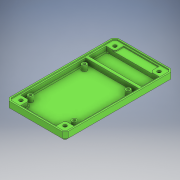
# Autodesk Inventor part: Case2
Saved by Autodesk Inventor 2020 (Build 240168000, 168)
## iProperties
Created: 2020-11-28
Part Number: Case2
Material: PBT Plastic
Document SubType Name: Modeling
Designer: Milosz
Density: 1.31 g/cm^3
Appearance: Smooth - White
Author: Milosz
## iProperties of the stored document _3DPrint.ipt
Created: 2020-11-29
Part Number: _3DPrint
Material: Generic
Document SubType Name: Modeling
Designer: Milosz
Density: 1 g/cm^3
Appearance: Default
Author: Milosz
Autodesk Inventor part; units mm, degrees
ref_plane "YZ Plane" through (0, 0, 0) normal (1, 0, 0) x (0, 1, 0)
ref_plane "XZ Plane" through (0, 0, 0) normal (0, 1, 0) x (-1, 0, 0)
ref_plane "XY Plane" through (0, 0, 0) normal (0, 0, 1) x (1, 0, 0)
sketch "Sketch4" plane through (0, 0, 0) normal (0, 1, 0) x (-1, 0, 0)
  circle A0 centre (-31.1, -7.3) radius 1.75
  line L0 (-34.858, -107.35) -> (16.858, -107.35)
  line L1 (16.858, -107.35) -> (18.95, -105.258)
  line L2 (18.95, -105.258) -> (18.95, -3.542)
  line L3 (18.95, -3.542) -> (16.858, -1.45)
  line L4 (16.858, -1.45) -> (-34.858, -1.45)
  line L5 (-34.858, -1.45) -> (-36.95, -3.542)
  line L6 (-36.95, -3.542) -> (-36.95, -105.258)
  line L7 (-36.95, -105.258) -> (-34.858, -107.35)
  circle A1 centre (-31.1, -101.5) radius 1.75
  circle A2 centre (13.1, -7.3) radius 1.75
  line L8 (8.7, -99.1) -> (10.7, -97.1)
  line L9 (8.7, -99.1) -> (8.7, -105.9)
  line L10 (8.7, -105.9) -> (-26.7, -105.9)
  line L11 (-26.7, -99.1) -> (-26.7, -105.9)
  line L12 (-28.7, -97.1) -> (-26.7, -99.1)
  line L13 (-35.5, -97.1) -> (-28.7, -97.1)
  line L14 (-35.5, -97.1) -> (-35.5, -11.7)
  line L15 (-35.5, -11.7) -> (-28.7, -11.7)
  line L16 (-26.7, -9.7) -> (-28.7, -11.7)
  line L17 (-26.7, -9.7) -> (-26.7, -2.9)
  line L18 (-26.7, -2.9) -> (8.7, -2.9)
  line L19 (8.7, -9.7) -> (8.7, -2.9)
  line L20 (10.7, -11.7) -> (8.7, -9.7)
  line L21 (17.5, -11.7) -> (10.7, -11.7)
  line L22 (17.5, -11.7) -> (17.5, -97.1)
  line L23 (17.5, -97.1) -> (10.7, -97.1)
  circle A3 centre (13.1, -101.5) radius 1.75
  line L24 (20.5, -2.9) -> (20.5, -105.9)
  line L25 (17.5, 0.1) -> (20.5, -2.9)
  line L26 (-35.5, 0.1) -> (17.5, 0.1)
  line L27 (-38.5, -2.9) -> (-35.5, 0.1)
  line L28 (-38.5, -105.9) -> (-38.5, -2.9)
  line L29 (-35.5, -108.9) -> (-38.5, -105.9)
  line L30 (17.5, -108.9) -> (-35.5, -108.9)
  line L31 (20.5, -105.9) -> (17.5, -108.9)
  line L32 (16.858, -107.35) -> (18.95, -105.258)
  line L33 (-34.858, -107.35) -> (16.858, -107.35)
  line L34 (-36.95, -105.258) -> (-34.858, -107.35)
  line L35 (-36.95, -3.542) -> (-36.95, -105.258)
  line L36 (-34.858, -1.45) -> (-36.95, -3.542)
  line L37 (16.858, -1.45) -> (-34.858, -1.45)
  line L38 (18.95, -3.542) -> (16.858, -1.45)
  line L39 (18.95, -105.258) -> (18.95, -3.542)
  line L40 (-37.05, -105.2994) -> (-37.05, -3.5006)
  line L41 (-37.05, -3.5006) -> (-34.8994, -1.35)
  line L42 (-34.8994, -1.35) -> (16.8994, -1.35)
  line L43 (16.8994, -1.35) -> (19.05, -3.5006)
  line L44 (19.05, -3.5006) -> (19.05, -105.2994)
  line L45 (19.05, -105.2994) -> (16.8994, -107.45)
  line L46 (16.8994, -107.45) -> (-34.8994, -107.45)
  line L47 (-34.8994, -107.45) -> (-37.05, -105.2994)
  point P0 (0, 0)
  point P1 (0, 0)
  dimension "d29" = 0.1
  constraints: 96 end point, 4 centre point, 7 other
  measures "d29" distance between parallel lines of L6 L40
extrude "Extrusion3" add sketch "Sketch4" along normal blind 1 contours L24 L31 L30 L29 L28 L27 L26 L25
extrude "Extrusion4" add sketch "Sketch4" against normal blind 5 contours L7 L6 L5 L4 L3 L2 L1 L0 | L24 L31 L30 L29 L28 L27 L26 L25 | L40 L41 L42 L43 L44 L45 L46 L47
sketch "Sketch5" plane through (0, -5, 0) normal (0, -1, 0) x (1, 0, 0)
  line L0 (38.5, -105.9) -> (38.5, -2.9) projected
  line L1 (38.5, -2.9) -> (35.5, 0.1) projected
  line L2 (35.5, 0.1) -> (-17.5, 0.1) projected
  line L3 (35.5, 0.1) -> (-17.5, 0.1) projected
  line L4 (-17.5, 0.1) -> (-20.5, -2.9) projected
  line L5 (-20.5, -2.9) -> (-20.5, -105.9) projected
  line L6 (-20.5, -105.9) -> (-17.5, -108.9) projected
  line L7 (-17.5, -108.9) -> (35.5, -108.9) projected
  line L8 (35.5, -108.9) -> (38.5, -105.9) projected
  line L9 (38.5, -105.9) -> (38.5, -2.9) projected
  line L10 (38.5, -2.9) -> (35.5, 0.1) projected
  circle A0 centre (31.1, -101.5) radius 1.75 projected
  circle A1 centre (-13.1, -101.5) radius 1.75 projected
  circle A2 centre (31.1, -7.3) radius 1.75 projected
  circle A3 centre (-13.1, -7.3) radius 1.75 projected
  line L11 (-17.5, -11.7) -> (-10.7, -11.7) projected
  line L12 (-10.7, -11.7) -> (-8.7, -9.7) projected
  line L13 (-8.7, -9.7) -> (-8.7, -2.9) projected
  line L14 (-8.7, -2.9) -> (26.7, -2.9) projected
  line L15 (26.7, -2.9) -> (26.7, -9.7) projected
  line L16 (26.7, -9.7) -> (28.7, -11.7) projected
  line L17 (28.7, -11.7) -> (35.5, -11.7) projected
  line L18 (35.5, -11.7) -> (35.5, -97.1) projected
  line L19 (35.5, -97.1) -> (28.7, -97.1) projected
  line L20 (28.7, -97.1) -> (26.7, -99.1) projected
  line L21 (26.7, -99.1) -> (26.7, -105.9) projected
  line L22 (26.7, -105.9) -> (-8.7, -105.9) projected
  line L23 (-8.7, -105.9) -> (-8.7, -99.1) projected
  line L24 (-8.7, -99.1) -> (-10.7, -97.1) projected
  line L25 (-10.7, -97.1) -> (-17.5, -97.1) projected
  line L26 (-17.5, -97.1) -> (-17.5, -11.7) projected
  point P0 (0, 0)
extrude "Extrusion5" add sketch "Sketch5" along normal blind 3 contours L8 L7 L6 L5 L4 L2 L1 L0 | L11 L12 L13 L14 L15 L16 L17 L18 L19 L20 L21 L22 L23 L24 L25 L26
sketch "Sketch6" plane through (0, -8, 0) normal (0, -1, 0) x (1, 0, 0)
  line L0 (38.5, -2.9) -> (35.5, 0.1) projected
  line L1 (35.5, 0.1) -> (-17.5, 0.1) projected
  line L2 (-17.5, 0.1) -> (-20.5, -2.9) projected
  line L3 (-20.5, -2.9) -> (-20.5, -105.9) projected
  line L4 (-20.5, -105.9) -> (-17.5, -108.9) projected
  line L5 (-17.5, -108.9) -> (35.5, -108.9) projected
  line L6 (35.5, -108.9) -> (38.5, -105.9) projected
  line L7 (38.5, -105.9) -> (38.5, -2.9) projected
  circle A0 centre (31.1, -101.5) radius 1.75 projected
  circle A1 centre (-13.1, -101.5) radius 1.75 projected
  circle A2 centre (31.1, -7.3) radius 1.75 projected
  circle A3 centre (-13.1, -7.3) radius 1.75 projected
  circle A4 centre (31.1, -7.3) radius 3
  circle A5 centre (31.1, -101.5) radius 3
  circle A6 centre (-13.1, -101.5) radius 3
  circle A7 centre (-13.1, -7.3) radius 3
  point P0 (0, 0)
  dimension "d17" = 6
  dimension "d18" = 6
  dimension "d19" = 6
  dimension "d20" = 6
  constraints: 4 centre point, 4 coincident
  measures "d17" diameter of A4
  measures "d18" diameter of A5
  measures "d19" diameter of A6
  measures "d20" diameter of A7
extrude "Extrusion6" cut sketch "Sketch6" against normal blind 6 contours A4 | A5 | A6 | A7
chamfer "Chamfer2" distance 1 angle 45 16 edges at (-17.5, -5, -54.4) (-9.7, -5, -98.1) (-8.7, -5, -102.5) (9, -5, -105.9) (26.7, -5, -102.5) (27.7, -5, -98.1) (35.5, -5, -54.4) (-14.1, -5, -11.7) (-9.7, -5, -10.7) (-8.7, -5, -6.3) (9, -5, -2.9) (26.7, -5, -6.3) (27.7, -5, -10.7) (32.1, -5, -11.7) (32.1, -5, -97.1) (-14.1, -5, -97.1)
chamfer "Chamfer3" distance 3 angle 45 8 edges at (38.5, -8, -54.4) (37, -8, -1.4) (9, -8, 0.1) (-19, -8, -1.4) (-20.5, -8, -54.4) (-19, -8, -107.4) (9, -8, -108.9) (37, -8, -107.4)
sketch "Sketch7" plane through (0, -5, 0) normal (0, 1, 0) x (1, 0, 0)
  line L0 (-13, 16.7) -> (31, 16.7) construction
  line L1 (31, 16.7) -> (31, 70.7) construction
  line L2 (31, 70.7) -> (-13, 70.7) construction
  line L3 (-13, 70.7) -> (-13, 16.7) construction
  circle A0 centre (-13, 70.7) radius 1.25
  circle A1 centre (31, 70.7) radius 1.25
  circle A2 centre (31, 16.7) radius 1.25
  circle A3 centre (-13, 16.7) radius 1.25
  line L4 (-13, 70.7) -> (31, 16.7) construction
  line L5 (-13, 16.7) -> (31, 70.7) construction
  line L6 (-16, 13.7) -> (34, 13.7) construction
  line L7 (34, 13.7) -> (34, 73.7) construction
  line L8 (34, 73.7) -> (-16, 73.7) construction
  line L9 (-16, 73.7) -> (-16, 13.7) construction
  line L10 (-16, 13.7) -> (34, 73.7) construction
  line L11 (34, 13.7) -> (-16, 73.7) construction
  line L12 (34.5, 96.1) -> (34.5, 12.7) construction
  line L13 (25.7, 98.6858) -> (28.2858, 96.1) construction
  line L14 (25.7, 104.9) -> (25.7, 98.6858) construction
  line L15 (-7.7, 104.9) -> (25.7, 104.9) construction
  line L16 (-7.7, 98.6858) -> (-7.7, 104.9) construction
  line L17 (-10.2858, 96.1) -> (-7.7, 98.6858) construction
  line L18 (-16.5, 12.7) -> (-16.5, 96.1) construction
  line L19 (-10.2858, 12.7) -> (-16.5, 12.7) construction
  line L20 (-7.7, 10.1142) -> (-10.2858, 12.7) construction
  line L21 (-7.7, 3.9) -> (-7.7, 10.1142) construction
  line L22 (25.7, 3.9) -> (-7.7, 3.9) construction
  line L23 (25.7, 10.1142) -> (25.7, 3.9) construction
  line L24 (28.2858, 12.7) -> (25.7, 10.1142) construction
  line L25 (34.5, 12.7) -> (28.2858, 12.7) construction
  line L26 (-7.7, 104.9) -> (25.7, 104.9) construction
  line L27 (9, 104.9) -> (9, 3.9) construction
  line L28 (25.7, 3.9) -> (-7.7, 3.9) construction
  circle A4 centre (-13, 70.7) radius 2.5
  circle A5 centre (31, 70.7) radius 2.5
  circle A6 centre (31, 16.7) radius 2.5
  circle A7 centre (-13, 16.7) radius 2.5
  line L29 (28.2858, 96.1) -> (34.5, 96.1) projected
  line L30 (-16.5, 96.1) -> (-10.2858, 96.1) projected
  point P0 (0, 0)
  point P1 (9, 43.7)
  point P2 (9, 43.7)
  dimension "d30" = 44
  dimension "d31" = 54
  dimension "d32" = 2.5
  dimension "d33" = 2.5
  dimension "d34" = 2.5
  dimension "d35" = 2.5
  dimension "d36" = 50
  dimension "d37" = 60
  dimension "d38" = 1
  dimension "d39" = 5
  dimension "d40" = 5
  dimension "d41" = 5
  dimension "d42" = 5
  constraints: 26 end point, 8 centre point, 8 coincident, 6 midpoint, 4 parallel, 2 horizontal, 2 perpendicular, 1 point on line
  measures "d30" distance of L2.end L1.end
  measures "d31" distance of L1.end L0.end
  measures "d32" diameter of A0
  measures "d33" diameter of A1
  measures "d34" diameter of A2
  measures "d35" diameter of A3
  measures "d36" distance of L8.end L7.end
  measures "d37" distance of L7.end L6.end
  measures "d38" distance between parallel lines of L25 L6
  measures "d39" diameter of A4
  measures "d40" diameter of A5
  measures "d41" diameter of A6
  measures "d42" diameter of A7
extrude "Extrusion7" add sketch "Sketch7" along normal blind 5
sketch "Sketch8" plane through (0, -5, 0) normal (0, 1, 0) x (1, 0, 0)
  line L0 (-14.5, 79.6) -> (35.5, 79.6)
  line L1 (35.5, 79.6) -> (35.5, 97.1)
  line L2 (35.5, 97.1) -> (-14.5, 97.1)
  line L3 (-14.5, 97.1) -> (-14.5, 79.6)
  line L4 (-14.5, 79.6) -> (35.5, 97.1) construction
  line L5 (35.5, 79.6) -> (-14.5, 97.1) construction
  circle A0 centre (31, 16.7) radius 2.5 projected
  circle A1 centre (31, 70.7) radius 2.5 projected
  circle A2 centre (-13, 16.7) radius 2.5 projected
  circle A3 centre (-13, 70.7) radius 2.5 projected
  line L6 (-16.5, 12.7) -> (-16.5, 96.1) projected
  line L7 (-10.2858, 12.7) -> (-16.5, 12.7) projected
  line L8 (-7.7, 10.1142) -> (-10.2858, 12.7) projected
  line L9 (-7.7, 3.9) -> (-7.7, 10.1142) projected
  line L10 (25.7, 3.9) -> (-7.7, 3.9) projected
  line L11 (25.7, 10.1142) -> (25.7, 3.9) projected
  line L12 (28.2858, 12.7) -> (25.7, 10.1142) projected
  line L13 (34.5, 12.7) -> (28.2858, 12.7) projected
  line L14 (34.5, 96.1) -> (34.5, 12.7) projected
  line L15 (25.7, 98.6858) -> (28.2858, 96.1) projected
  line L16 (25.7, 104.9) -> (25.7, 98.6858) projected
  line L17 (-7.7, 104.9) -> (25.7, 104.9) projected
  line L18 (-7.7, 98.6858) -> (-7.7, 104.9) projected
  line L19 (-10.2858, 96.1) -> (-7.7, 98.6858) projected
  line L20 (28.7, 97.1) -> (35.5, 97.1) projected
  line L21 (35.5, 97.1) -> (35.5, 11.7) projected
  line L22 (28.2858, 96.1) -> (34.5, 96.1) projected
  line L23 (-16.5, 96.1) -> (-10.2858, 96.1) projected
  line L24 (26.7, 105.9) -> (-8.7, 105.9) projected
  line L25 (-7.7, 104.9) -> (-8.7, 105.9) projected
  line L26 (-7.7, 104.9) -> (25.7, 104.9) projected
  line L27 (25.7, 104.9) -> (26.7, 105.9) projected
  line L28 (-8.7, 105.9) -> (-8.7, 99.1) projected
  line L29 (-7.7, 98.6858) -> (-8.7, 99.1) projected
  line L30 (-7.7, 98.6858) -> (-7.7, 104.9) projected
  line L31 (-7.7, 104.9) -> (-8.7, 105.9) projected
  line L32 (-8.7, 99.1) -> (-10.7, 97.1) projected
  line L33 (-10.2858, 96.1) -> (-10.7, 97.1) projected
  line L34 (-10.2858, 96.1) -> (-7.7, 98.6858) projected
  line L35 (-7.7, 98.6858) -> (-8.7, 99.1) projected
  line L36 (28.7, 97.1) -> (26.7, 99.1) projected
  line L37 (25.7, 98.6858) -> (26.7, 99.1) projected
  line L38 (25.7, 98.6858) -> (28.2858, 96.1) projected
  line L39 (28.2858, 96.1) -> (28.7, 97.1) projected
  line L40 (26.7, 99.1) -> (26.7, 105.9) projected
  line L41 (25.7, 104.9) -> (26.7, 105.9) projected
  line L42 (25.7, 104.9) -> (25.7, 98.6858) projected
  line L43 (25.7, 98.6858) -> (26.7, 99.1) projected
  point P0 (0, 0)
  point P1 (10.5, 88.35)
  point P2 (34.5, 97.1)
  point P3 (-9.2858, 97.1)
  point P4 (-14.5, 96.1)
  dimension "d47" = 50
  dimension "d48" = 17.5
  constraints: 12 end point, 2 collinear, 2 midpoint, 2 parallel, 1 horizontal, 1 perpendicular
  measures "d47" distance of L2.end L1.end
  measures "d48" distance of L1.end L0.end
extrude "Extrusion8" cut sketch "Sketch8" along normal blind 5 contours L3 L23 L19 L2 L15 L22 L14 L0 | L14 L22 L39 L2 L1 L0 | L3 L2 L33 L23 | L33 L2 L19 | L15 L2 L39
extrude "Extrusion9" add sketch "Sketch8" along normal blind 4 contours L32 L29 L19 L2 | L19 L18 L17 L16 L15 L2 | L2 L15 L37 L36 | L28 L25 L18 L29 | L37 L16 L27 L40 | L24 L27 L17 L25
sketch "Sketch9" plane through (0, -5, 0) normal (0, 1, 0) x (1, 0, 0)
  line L0 (34.5, 79.6) -> (35.5, 79.6) projected
  line L1 (-17.5, 97.1) -> (-17.5, 11.7) projected
  line L2 (35.5, 79.6) -> (-17.5, 79.6)
  line L3 (-17.5, 79.6) -> (-17.5, 76.6)
  line L4 (-17.5, 76.6) -> (35.5, 76.6)
  line L5 (35.5, 76.6) -> (35.5, 79.6)
  point P0 (0, 0)
  dimension "d53" = 3
  constraints: 8 end point, 2 parallel, 1 horizontal, 1 perpendicular, 1 point on line
  measures "d53" distance of L3.end L2.end
extrude "Extrusion10" add sketch "Sketch9" along normal blind 5
equation "\"d18\" = d17"
equation "\"d19\" = d17"
equation "\"d20\" = d17"
equation "\"d33\" = d32"
equation "\"d34\" = d32"
equation "\"d35\" = d32"
equation "\"d43\" = d42"
body "Solid2"
